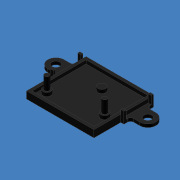
# Autodesk Inventor part: Spike Bottom Cover
Saved by Autodesk Inventor 2012 (Build 160160000, 160)
## iProperties
Shininess: 64.0
Length Units: 11269
Angle Units: 11279
Time Units: 11290
Mass Units: 11283
Length Display Precision: 3
Angle Display Precision: 2
Compacted: True
Part Number: Spike Bottom Cover
Document SubType Name: Modeling
Created: 2006-01-06
Material: ABS Plastic
Designer: Owner
Density: 1 g/cm^3
Density: 0.0
Volumn: 0.0
Area: 0.0
PropertySet Name: Model Information
Control State: 0
Master: False
Checked Out: False
Author: Owner
Autodesk Inventor part; units mm, degrees
ref_plane "YZ Plane" through (0, 0, 0) normal (1, 0, 0) x (0, 1, 0)
ref_plane "XZ Plane" through (0, 0, 0) normal (0, 1, 0) x (-1, 0, 0)
ref_plane "XY Plane" through (0, 0, 0) normal (0, 0, 1) x (1, 0, 0)
sketch "Sketch1" plane through (0, 0, 0) normal (0, 0, 1) x (1, 0, 0)
  line L0 (-21.5, 19) -> (21.5, 19)
  line L1 (21.5, 19) -> (21.5, -19)
  line L2 (21.5, -19) -> (-21.5, -19)
  line L3 (-21.5, -19) -> (-21.5, 19)
  line L4 (0, 0) -> (0, 19) construction
  line L5 (0, 0) -> (0, -19) construction
  line L6 (0, 0) -> (21.5, 0) construction
  line L7 (0, 0) -> (-21.5, 0) construction
  dimension "d0" = 43
  dimension "d1" = 38
  constraints: 16 end point, 4 midpoint, 3 horizontal, 2 collinear, 2 parallel, 2 vertical, 1 perpendicular, 1 other
  measures "d0" distance of L0.start L0.end
  measures "d1" distance of L2.end L0.start
extrude "Extrusion1" add sketch "Sketch1" along normal blind 4.5
sketch "Sketch2" plane through (0, 0, 4.5) normal (0, 0, 1) x (1, 0, 0)
  line L0 (21.5, 19) -> (21.5, -19) projected
  line L1 (-21.5, 19) -> (21.5, 19) projected
  line L2 (-21.5, -19) -> (-21.5, 19) projected
  line L3 (21.5, -19) -> (-21.5, -19) projected
  line L4 (19.7, 17.2) -> (19.7, -17.2)
  line L5 (19.7, -17.2) -> (-19.7, -17.2)
  line L6 (-19.7, -17.2) -> (-19.7, 17.2)
  line L7 (-19.7, 17.2) -> (19.7, 17.2)
  dimension "d4" = 1.8
  constraints: 8 end point, 3 other
  measures "d4" distance between parallel lines of L1 L7
extrude "Extrusion2" cut sketch "Sketch2" against normal blind 2.25 contours L4 L5 L6 L7
sketch "Sketch3" plane through (0, 0, 0) normal (0, 0, -1) x (-1, 0, 0)
  line L0 (21.5, 19) -> (-21.5, 19) projected
  line L1 (-21.5, 19) -> (-21.5, -19) projected
  line L2 (-21.5, 17) -> (-23.5, 17)
  line L3 (-23.5, 17) -> (-23.5, 12.725)
  line L4 (-23.5, 12.725) -> (-34.5, 12.725)
  line L5 (-34.5, 12.725) -> (-34.5, 2.425)
  line L6 (-34.5, 2.425) -> (-23.5, 2.425)
  line L7 (-23.5, 2.425) -> (-23.5, -1.85)
  line L8 (-23.5, -1.85) -> (-21.5, -1.85)
  dimension "d7" = 2
  dimension "d8" = 2
  dimension "d9" = 18.85
  dimension "d10" = 10.3
  dimension "d11" = 13
  constraints: 14 end point, 4 horizontal, 3 equal length, 3 vertical, 2 point on line, 1 collinear
  measures "d7" distance from line of L2.start L0
  measures "d8" distance of L7.end L8.end
  measures "d9" distance between parallel lines of L8 L2
  measures "d10" distance of L4.end L5.end
  measures "d11" distance between parallel lines of L5 L1
extrude "Extrusion3" add sketch "Sketch3" against normal blind 2
fillet "Fillet1" radius 5.15 2 edges at (34.5, 2.425, 1) (34.5, 12.725, 1)
fillet "Fillet1" radius 2 2 edges at (23.5, 2.425, 1) (23.5, 12.725, 1)
sketch "Sketch4" plane through (0, 0, 2) normal (0, 0, 1) x (1, 0, 0)
  arc A0 (29.35, 2.425) -> (29.35, 12.725) centre (29.35, 7.575) ccw projected
  constraints: 1 coincident
hole "Hole1" at (29.35, 7.575, 2) direction (0, 0, -1) diameter 5 end through all
sketch "Sketch5" plane through (0, 0, 2) normal (0, 0, 1) x (1, 0, 0)
  line L0 (21.5, -1.85) -> (21.5, 17) projected
  line L1 (23.5, -1.85) -> (21.5, -1.85)
  line L2 (21.5, -1.85) -> (21.5, -0.5)
  line L3 (21.5, -0.5) -> (23.5, -0.5)
  line L4 (23.5, -0.5) -> (23.5, -1.85)
  line L5 (23.5, 17) -> (21.5, 17)
  line L6 (21.5, 17) -> (21.5, 15.65)
  line L7 (21.5, 15.65) -> (23.5, 15.65)
  line L8 (23.5, 15.65) -> (23.5, 17)
  dimension "d23" = 1.35
  constraints: 16 end point, 4 parallel, 2 horizontal, 2 perpendicular, 2 point on line, 1 collinear
  measures "d23" distance of L3.end L1.start
extrude "Extrusion4" add sketch "Sketch5" along normal blind 5.15
mirror "Mirror1" about plane through (0, 0, 0) normal (1, 0, 0) of "Extrusion4", "Hole1", "Extrusion3", "Fillet1"
sketch "Sketch6" plane through (0, 0, 2.25) normal (0, 0, 1) x (1, 0, 0)
  circle A0 centre (0, 7.575) radius 2.5
  line L0 (-21.5, 19) -> (21.5, 19) projected
  circle A1 centre (-29.35, 7.575) radius 2.5 projected
  point P0 (0, 0)
  dimension "d26" = 5
  constraints: 1 centre point, 1 horizontal alignment, 1 vertical alignment, 1 other
  measures "d26" diameter of A0
extrude "Extrusion5" add sketch "Sketch6" along normal up to surface (2.25 mm away) contours A0
sketch "Sketch7" plane through (0, 0, 2.25) normal (0, 0, 1) x (1, 0, 0)
  circle A0 centre (-15.9, -11.65) radius 2.5
  circle A1 centre (15.4, -6) radius 2.5
  line L0 (-21.5, -19) -> (-21.5, -1.85) projected
  line L1 (21.5, -19) -> (-21.5, -19) projected
  line L2 (21.5, -1.85) -> (21.5, -19) projected
  dimension "d30" = 5
  dimension "d31" = 5.6
  dimension "d32" = 7.35
  dimension "d33" = 6.1
  dimension "d34" = 13
  constraints: 2 centre point, 1 equal radius
  measures "d30" diameter of A0
  measures "d31" distance from line of A0.centre L0
  measures "d32" distance from line of L1 A0.centre
  measures "d33" distance from line of L2 A1.centre
  measures "d34" distance from line of L1 A1.centre
extrude "Extrusion6" add sketch "Sketch7" along normal up to surface (2.25 mm away)
sketch "Sketch8" plane through (-15.9, -11.65, 4.5) normal (0, 0, 1) x (1, 0, 0)
  circle A0 centre (0, 0) radius 2.5 projected
  circle A1 centre (0, 0) radius 1.5
  circle A2 centre (31.3, 5.65) radius 2.5 projected
  circle A3 centre (31.3, 5.65) radius 1.5
  dimension "d37" = 3
  constraints: 2 centre point, 2 coincident, 2 concentric, 1 equal radius
  measures "d37" diameter of A1
extrude "Extrusion7" add sketch "Sketch8" along normal blind 8 contours A1 | A3
body "Solid1"
